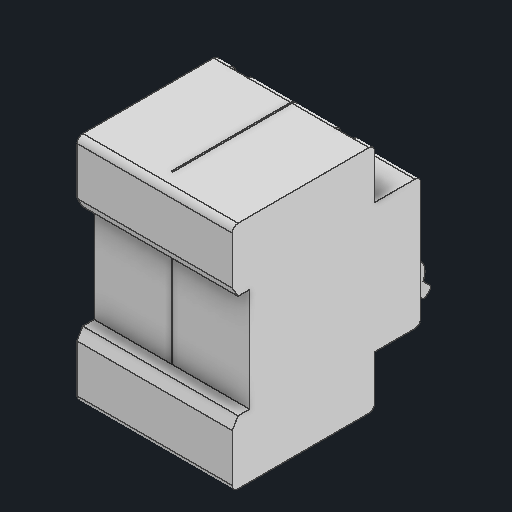
# Autodesk Inventor part: DIHOOL-DZ47Z-120-1000V-100A
Saved by Autodesk Inventor 2025.2 (Build 292293000, 293)
## iProperties
Created: 2025-11-01
Part Number: DIHOOL-DZ47Z-120-1000V-100A
Material: Generic
Document SubType Name: Modeling
Designer: valer
Density: 1 g/cm^3
Appearance: Default
Author: valer
Autodesk Inventor part; units mm, degrees
sketch "Base" plane through (0, 0, 0) normal (0, 0, 1) x (1, 0, 0)
  line L0 (-27, -40) -> (27, -40)
  line L1 (27, -40) -> (27, 40)
  line L2 (27, 40) -> (-27, 40)
  line L3 (-27, 40) -> (-27, -40)
  line L4 (-27, -40) -> (27, 40) construction
  line L5 (27, -40) -> (-27, 40) construction
  point P0 (0, 0)
  dimension "d0" = 54
  dimension "d1" = 80
  constraints: 12 end point, 2 midpoint, 2 parallel, 1 horizontal, 1 perpendicular
  measures "d0" distance of L1.end L2.end
  measures "d1" distance of L0.end L1.end
extrude "BaseFeature" add sketch "Base" along normal blind 49.5
sketch "Sketch3" plane through (-27, -40, 0) normal (-1, 0, 0) x (0, 0, 1)
  line L0 (49.5, 0) -> (49.5, 80) projected
  line L1 (49.5, 18.5359) -> (47.5, 22)
  line L2 (47.5, 22) -> (43.5, 22)
  line L3 (43.5, 22) -> (43.5, 40)
  line L4 (0, 40) -> (49.5, 40) construction
  line L5 (49.5, 61.4641) -> (47.5, 58)
  line L6 (47.5, 58) -> (43.5, 58)
  line L7 (43.5, 40) -> (43.5, 58)
  dimension "d4" = 6
  dimension "d5" = 18
  dimension "d6" = 30
  dimension "d7" = 2
  constraints: 14 end point, 3 symmetric about line, 2 perpendicular, 2 point on line, 1 midpoint, 1 vertical
  measures "d4" distance between parallel lines of L0 L3
  measures "d5" distance from line of L4 L1.end
  measures "d6" angle of L0 L1
  measures "d7" distance from line of L0 L1.end
extrude "Extrusion2" cut sketch "Sketch3" against normal through all
fillet "Fillet1" radius 2 4 edges at (0, -40, 49.5) (0, 40, 49.5) (0, -40, 0) (0, 40, 0)
sketch "Sketch5" plane through (27, -18, 43.5) normal (1, 0, 0) x (0, 0, -1)
  line L0 (43.5, -20) -> (43.5, 56) projected
  line L1 (43.5, -4.5) -> (59.5, -4.5)
  line L2 (59.5, -4.5) -> (59.5, 40.5)
  line L3 (59.5, 40.5) -> (43.5, 40.5)
  line L4 (43.5, 40.5) -> (43.5, -4.5)
  line L5 (43.5, 18) -> (59.5, 18) construction
  line L6 (43.5, 56) -> (43.5, -20) projected
  point P0 (51.5, 40.5)
  dimension "d11" = 45
  dimension "d12" = 16
  constraints: 10 end point, 2 midpoint, 2 parallel, 2 perpendicular, 1 horizontal, 1 point on line
  measures "d11" distance from line of point (51.5, 40.5) L1
  measures "d12" distance of L1.start L1.end
extrude "Extrusion3" add sketch "Sketch5" against normal up to surface (54 mm away)
fillet "Fillet2" radius 2 2 edges at (0, -22.5, -16) (0, 22.5, -16)
sketch "Sketch6" plane through (27, -20.5, -16) normal (0, 0, -1) x (-1, 0, 0)
  line L0 (54, 60.5) -> (0, 60.5) construction
  line L1 (27, 60.5) -> (27, -19.5) construction
  line L2 (54, -19.5) -> (0, -19.5) construction
  line L3 (26.75, -19.5) -> (26.75, 60.5)
  line L4 (26.75, 60.5) -> (27.25, 60.5)
  line L5 (27.25, 60.5) -> (27.25, -19.5)
  line L6 (27.25, -19.5) -> (26.75, -19.5)
  line L7 (26.75, -19.5) -> (27.25, 60.5) construction
  line L8 (26.75, 60.5) -> (27.25, -19.5) construction
  point P0 (27, 20.5)
  dimension "d16" = 0.5
  constraints: 14 end point, 4 midpoint, 2 parallel, 2 perpendicular
  measures "d16" distance between parallel lines of L3 L5
extrude "Extrusion4" cut sketch "Sketch6" against normal up to surface (59.5 mm away)
sketch "Sketch7" plane through (0, 0, 0) normal (0, 0, -1) x (-1, 0, 0)
  line L0 (-27, 40) -> (27, 40) projected
  line L1 (-27, 38) -> (-0.25, 38) projected
  line L2 (-21.5, 40) -> (-15, 40)
  line L3 (-15, 40) -> (-15, 38)
  line L4 (-15, 38) -> (-21.5, 38)
  line L5 (-21.5, 38) -> (-21.5, 40)
  line L6 (-24.7, 38) -> (-11.8, 38)
  line L7 (-11.8, 38) -> (-11.8, 28)
  line L8 (-11.8, 28) -> (-24.7, 28)
  line L9 (-24.7, 28) -> (-24.7, 38)
  line L10 (-27, 38) -> (-27, 40) projected
  line L11 (-18.25, 28) -> (-18.25, 40) construction
  line L12 (-27, 22.5) -> (-27, 38) projected
  line L13 (37.8, 0) -> (-37.8, 0) construction
  line L14 (0, -56) -> (0, 56) construction
  line L15 (15, 40) -> (15, 38)
  line L16 (21.5, 38) -> (21.5, 40)
  line L17 (24.7, 38) -> (11.8, 38)
  line L18 (11.8, 28) -> (24.7, 28)
  line L19 (24.7, 28) -> (24.7, 38)
  line L20 (11.8, 28) -> (11.8, 38)
  line L21 (-15, -40) -> (-15, -38)
  line L22 (-21.5, -38) -> (-21.5, -40)
  line L23 (-24.7, -38) -> (-11.8, -38)
  line L24 (-11.8, -38) -> (-11.8, -28)
  line L25 (-11.8, -28) -> (-24.7, -28)
  line L26 (-24.7, -28) -> (-24.7, -38)
  line L27 (24.7, -28) -> (24.7, -38)
  line L28 (11.8, -28) -> (24.7, -28)
  line L29 (24.7, -38) -> (11.8, -38)
  line L30 (15, -40) -> (15, -38)
  line L31 (21.5, -38) -> (21.5, -40)
  line L32 (11.8, -28) -> (11.8, -38)
  line L33 (-27, -40) -> (-0.25, -40) projected
  line L34 (0.25, -40) -> (27, -40) projected
  point P0 (0, 0)
  point P1 (-21.5, 39)
  dimension "d19" = 5.5
  dimension "d20" = 6.5
  dimension "d21" = 2.3
  dimension "d22" = 10
  constraints: 54 end point, 24 symmetric about line, 4 parallel, 3 midpoint, 3 perpendicular, 3 point on line, 2 horizontal, 1 vertical
  measures "d19" distance from line of L10 point (-21.5, 39)
  measures "d20" distance between parallel lines of L3 L5
  measures "d21" distance between parallel lines of L12 L9
  measures "d22" distance between parallel lines of L8 L6
extrude "Extrusion5" cut sketch "Sketch7" against normal blind 2 contours L0 L3 L1 L5 | L1 L7 L8 L9 | L0 L16 L17 L15 | L17 L19 L18 L20 | L33 L22 L23 L21 | L23 L26 L25 L24 | L27 L29 L32 L28 | L31 L34 L30 L29
sketch "Sketch8" plane through (0, 0, 2) normal (0, 0, -1) x (-1, 0, 0)
  line L0 (-24.7, 28) -> (-24.7, 38) projected
  line L1 (-11.8, 28) -> (-24.7, 28) projected
  line L2 (-24.7, 38) -> (-11.8, 28) construction
  line L3 (-11.8, 38) -> (-0.25, 38) projected
  line L4 (-24.7, 28) -> (-11.8, 38) construction
  circle A0 centre (-18.25, 33) radius 3
  line L5 (37.8, 0) -> (-37.8, 0) projected
  line L6 (0, -56) -> (0, 56) projected
  circle A1 centre (18.25, 33) radius 3
  circle A2 centre (-18.25, -33) radius 3
  circle A3 centre (18.25, -33) radius 3
  point P0 (0, 0)
  dimension "d25" = 6
  constraints: 4 centre point, 4 end point, 3 symmetric about line, 1 midpoint, 3 other
  measures "d25" diameter of A0
extrude "Extrusion6" cut sketch "Sketch8" against normal blind 2
ref_plane "Work Plane1" through (25.5, -18, 43.5) normal (1, 0, 0) x (0, 0, -1)
ref_plane "Work Plane2" through (1.75, -20.5, -16) normal (-1, 0, 0) x (0, 0, 1)
sketch "Sketch9" plane through (25.5, -18, 43.5) normal (1, 0, 0) x (0, 0, -1)
  circle A0 centre (56.5, 9.5) radius 6
  line L0 (43.5, -4.5) -> (57.5, -4.5) projected
  line L1 (50.5, 15.5) -> (62.5, 15.5) construction
  line L2 (62.5, 15.5) -> (62.5, 3.5) construction
  line L3 (62.5, 3.5) -> (50.5, 3.5) construction
  line L4 (50.5, 3.5) -> (50.5, 15.5) construction
  line L5 (50.5, 15.5) -> (62.5, 3.5) construction
  line L6 (62.5, 15.5) -> (50.5, 3.5) construction
  line L7 (59.5, -2.5) -> (59.5, 38.5) projected
  point P0 (43.5, 18)
  point P1 (59.5, 14.6962)
  point P2 (59.5, 4.3038)
  dimension "d30" = 12
  dimension "d31" = 14
  dimension "d32" = 8
  dimension "d33" = 3
  constraints: 12 end point, 2 midpoint, 2 parallel, 2 tangent, 1 centre point, 1 horizontal, 1 perpendicular
  measures "d30" diameter of A0
  measures "d31" distance from line of L0 A0.centre
  measures "d32" distance between parallel lines of L0 L3
  measures "d33" distance between parallel lines of L7 L2
extrude "Extrusion7" add sketch "Sketch9" against normal up to surface (23.75 mm away) contours A0 L7 picked at (60.5, 9.5)
ref_plane "Work Plane3" through (23.5, -18, 43.5) normal (1, 0, 0) x (0, 0, -1)
ref_plane "Work Plane4" through (3.75, -8.5, -13) normal (-1, 0, 0) x (0, 0, 1)
sketch "Sketch10" plane through (23.5, -18, 43.5) normal (1, 0, 0) x (0, 0, -1)
  arc A0 (59.5, 4.3038) -> (59.5, 14.6962) centre (56.5, 9.5) ccw projected
  arc A1 (59.25, 4.7369) -> (59.25, 14.2631) centre (56.5, 9.5) ccw
  line L0 (59.5, 14.6962) -> (59.5, 14.1098)
  line L1 (59.5, -2.5) -> (59.5, 38.5) projected
  line L2 (59.5, 4.3038) -> (59.5, 4.8902)
  point P0 (43.5, 18)
  point P1 (59.5, 4.8902)
  dimension "d38" = 0.5
  constraints: 4 end point, 4 point on circle, 2 point on line, 1 centre point
  measures "d38" radial gap between concentric circles of A0 A1
extrude "Extrusion8" cut sketch "Sketch10" against normal up to surface (19.75 mm away) contours L1 A1 L0 A0
ref_plane "Work Plane5" through (19.5, -18, 43.5) normal (-1, 0, 0) x (0, 0, 1)
ref_plane "Work Plane6" through (7.75, -8.5, -13) normal (1, 0, 0) x (0, 0, -1)
sketch "Sketch12" plane through (7.75, -8.5, -13) normal (1, 0, 0) x (0, 0, -1)
  arc A0 (3, -4.6098) -> (3, 4.6098) centre (0, 0) ccw projected
  arc A1 (2.7273, -4.1907) -> (2.7273, 4.1907) centre (0, 0) ccw
  line L0 (3, 4.6098) -> (3, 4)
  line L1 (3, -12) -> (3, 29) projected
  line L2 (3, -4.6098) -> (3, -4)
  point P0 (-13, 8.5)
  dimension "d43" = 0.5
  constraints: 4 end point, 4 point on circle, 2 point on line, 1 centre point
  measures "d43" radial gap between concentric circles of A0 A1
extrude "Extrusion9" cut sketch "Sketch12" along normal up to surface (11.75 mm away) contours L1 A1 L0 A0
mirror "Mirror1" about plane through (0, 0, 0) normal (1, 0, 0) of "Extrusion7", "Extrusion8", "Extrusion9"
sketch "Sketch13" plane through (27, -20.5, -16) normal (0, 0, -1) x (-1, 0, 0)
  line L0 (1.5, 17.1962) -> (3.5, 17.1962) construction
  line L1 (3.5, 17.1962) -> (3.5, 16.6098) construction
  line L2 (3.5, 16.6098) -> (7.5, 16.6098) construction
  line L3 (7.5, 16.6098) -> (7.5, 16) construction
  line L4 (19.25, 16) -> (7.5, 16) construction
  line L5 (19.25, 16.6098) -> (19.25, 16) construction
  line L6 (19.25, 16.6098) -> (23.25, 16.6098) construction
  line L7 (23.25, 17.1962) -> (23.25, 16.6098) construction
  line L8 (23.25, 17.1962) -> (25.25, 17.1962) construction
  line L9 (25.25, 17.1962) -> (25.25, 6.8038) construction
  line L10 (25.25, 6.8038) -> (23.25, 6.8038) construction
  line L11 (23.25, 7.3902) -> (23.25, 6.8038) construction
  line L12 (19.25, 7.3902) -> (23.25, 7.3902) construction
  line L13 (19.25, 8) -> (19.25, 7.3902) construction
  line L14 (19.25, 8) -> (7.5, 8) construction
  line L15 (7.5, 8) -> (7.5, 7.3902) construction
  line L16 (3.5, 7.3902) -> (7.5, 7.3902) construction
  line L17 (3.5, 7.3902) -> (3.5, 6.8038) construction
  line L18 (3.5, 6.8038) -> (1.5, 6.8038) construction
  line L19 (1.5, 6.8038) -> (1.5, 17.1962) construction
  line L20 (26.75, 0) -> (26.75, 41) construction
  line L21 (0, 41) -> (26.75, 41) construction
  line L22 (0, 0) -> (0, 41) construction
  line L23 (26.75, 0) -> (0, 0) construction
  line L24 (28.75, 17.1962) -> (30.75, 17.1962) construction
  line L25 (30.75, 17.1962) -> (30.75, 16.6098) construction
  line L26 (34.75, 16.6098) -> (30.75, 16.6098) construction
  line L27 (34.75, 16.6098) -> (34.75, 16) construction
  line L28 (34.75, 16) -> (46.5, 16) construction
  line L29 (46.5, 16.6098) -> (46.5, 16) construction
  line L30 (50.5, 16.6098) -> (46.5, 16.6098) construction
  line L31 (50.5, 17.1962) -> (50.5, 16.6098) construction
  line L32 (50.5, 17.1962) -> (52.5, 17.1962) construction
  line L33 (52.5, 17.1962) -> (52.5, 6.8038) construction
  line L34 (52.5, 6.8038) -> (50.5, 6.8038) construction
  line L35 (50.5, 7.3902) -> (50.5, 6.8038) construction
  line L36 (50.5, 7.3902) -> (46.5, 7.3902) construction
  line L37 (46.5, 8) -> (46.5, 7.3902) construction
  line L38 (34.75, 8) -> (46.5, 8) construction
  line L39 (34.75, 8) -> (34.75, 7.3902) construction
  line L40 (34.75, 7.3902) -> (30.75, 7.3902) construction
  line L41 (30.75, 7.3902) -> (30.75, 6.8038) construction
  line L42 (30.75, 6.8038) -> (28.75, 6.8038) construction
  line L43 (28.75, 6.8038) -> (28.75, 17.1962) construction
  line L44 (27.25, 41) -> (27.25, 0) construction
  line L45 (54, 0) -> (27.25, 0) construction
  line L46 (54, 0) -> (54, 41) construction
  line L47 (27.25, 41) -> (54, 41) construction
  line L48 (26.75, 23.6962) -> (18.75, 23.6962)
  line L49 (18.75, 23.6962) -> (18.75, 26.6962)
  line L50 (18.75, 26.6962) -> (26.75, 26.6962)
  line L51 (26.75, 26.6962) -> (26.75, 23.6962)
  line L52 (54, 23.6962) -> (46, 23.6962)
  line L53 (46, 23.6962) -> (46, 26.6962)
  line L54 (46, 26.6962) -> (54, 26.6962)
  line L55 (54, 26.6962) -> (54, 23.6962)
  point P0 (27, 20.5)
  dimension "d46" = 8
  dimension "d47" = 6.5
  dimension "d48" = 3
  constraints: 16 end point, 4 parallel, 2 equal length, 2 horizontal, 2 perpendicular, 2 point on line, 1 collinear
  measures "d46" distance of L49.end L50.end
  measures "d47" distance from line of L8.end L48
  measures "d48" distance between parallel lines of L48 L50
extrude "Extrusion10" cut sketch "Sketch13" against normal blind 0.5
sketch "Sketch14" plane through (0, 0, 0) normal (1, 0, 0) x (0, 1, 0)
  arc A0 (-13.6962, -16) -> (-3.3038, -16) centre (-8.5, -13) ccw projected
  line L0 (-8.5, -13) -> (-15.5711, -20.0711) construction
  line L1 (-20.5, -16) -> (20.5, -16) projected
  line L2 (-9.8258, -11.6742) -> (-16.8969, -18.7452)
  line L3 (-16.8969, -18.7452) -> (-14.2452, -21.3969)
  line L4 (-14.2452, -21.3969) -> (-7.1742, -14.3258)
  line L5 (-7.1742, -14.3258) -> (-9.8258, -11.6742)
  line L6 (-9.8258, -11.6742) -> (-14.2452, -21.3969) construction
  line L7 (-16.8969, -18.7452) -> (-7.1742, -14.3258) construction
  point P0 (0, 0)
  point P1 (-12.0355, -16.5355)
  point P2 (-11.2043, -18.356)
  point P3 (-14.1517, -16)
  dimension "d51" = 45
  dimension "d52" = 10
  dimension "d53" = 3.75
  constraints: 14 end point, 4 midpoint, 3 parallel, 1 perpendicular
  measures "d51" angle of L1 L0
  measures "d52" distance of L0.end L0.start
  measures "d53" distance of L2.end L3.end
extrude "Extrusion11" add sketch "Sketch14" along normal up to surface (25.5 mm away) contours A0 L4 L3 L2 L1
fillet "Fillet3" radius 1 2 edges at (12.75, -14.2452, -21.3969) (12.75, -16.8969, -18.7452)
mirror "Mirror2" about plane through (0, 0, 0) normal (1, 0, 0) of "Fillet3", "Extrusion11"
body "Solid1"
